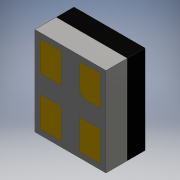
# Autodesk Inventor part: LXDC2HN18A-097
Saved by Autodesk Inventor 2016 (Build 200138000, 138)
## iProperties
Created: 2016-07-07
Part Number: LXDC2HN18A-097
Material: Generic
Document SubType Name: Modeling
Designer: Jonathan
Density: 1 g/cm^3
Appearance: Default
Author: Jonathan
Autodesk Inventor part; units mm, degrees
ref_plane "YZ Plane" through (0, 0, 0) normal (1, 0, 0) x (0, 1, 0)
ref_plane "XZ Plane" through (0, 0, 0) normal (0, 1, 0) x (-1, 0, 0)
ref_plane "XY Plane" through (0, 0, 0) normal (0, 0, 1) x (1, 0, 0)
sketch "Sketch1" plane through (0, 0, 0) normal (0, 1, 0) x (-1, 0, 0)
  line L0 (-1, 1.25) -> (1, 1.25)
  line L1 (1, 1.25) -> (1, -1.25)
  line L2 (1, -1.25) -> (-1, -1.25)
  line L3 (-1, -1.25) -> (-1, 1.25)
  line L4 (-1, 1.25) -> (1, -1.25) construction
  line L5 (1, 1.25) -> (-1, -1.25) construction
  point P0 (0, 0)
  dimension "d0" = 2
  dimension "d1" = 2.5
  constraints: 12 end point, 2 midpoint, 2 parallel, 1 horizontal, 1 perpendicular
  measures "d0" distance of L1.end L2.end
  measures "d1" distance of L0.end L1.end
extrude "Extrusion1" add sketch "Sketch1" along normal blind 0.6
sketch "Sketch2" plane through (0, 0.6, 0) normal (0, 1, 0) x (1, 0, 0)
  line L0 (-1, 1.25) -> (-1, -1.25) projected
  line L1 (-1, -1.25) -> (1, -1.25) projected
  line L2 (1, -1.25) -> (1, 1.25) projected
  line L3 (1, 1.25) -> (-1, 1.25) projected
  point P0 (0, 0)
extrude "Extrusion2" add sketch "Sketch2" along normal blind 0.5 separate body
sketch "Sketch3" plane through (0, 0, 0) normal (0, -1, 0) x (1, 0, 0)
  line L0 (0.85, 1.1) -> (0.25, 1.1)
  line L1 (0.25, 1.1) -> (0.25, 0.3914)
  line L2 (0.3914, 0.25) -> (0.85, 0.25)
  line L3 (0.85, 0.25) -> (0.85, 1.1)
  line L4 (-0.25, 1.1) -> (-0.85, 1.1)
  line L5 (-0.85, 1.1) -> (-0.85, 0.25)
  line L6 (-0.85, 0.25) -> (-0.25, 0.25)
  line L7 (-0.25, 0.25) -> (-0.25, 1.1)
  line L8 (-0.25, -0.25) -> (-0.85, -0.25)
  line L9 (-0.85, -0.25) -> (-0.85, -1.1)
  line L10 (-0.85, -1.1) -> (-0.25, -1.1)
  line L11 (-0.25, -1.1) -> (-0.25, -0.25)
  line L12 (0.85, -0.25) -> (0.25, -0.25)
  line L13 (0.25, -0.25) -> (0.25, -1.1)
  line L14 (0.25, -1.1) -> (0.85, -1.1)
  line L15 (0.85, -1.1) -> (0.85, -0.25)
  line L16 (0.3914, 0.25) -> (0.25, 0.3914)
  line L17 (1, 1.25) -> (-1, 1.25) projected
  line L18 (-1, 1.25) -> (-1, -1.25) projected
  line L19 (-1, -1.25) -> (1, -1.25) projected
  line L20 (1, -1.25) -> (1, 1.25) projected
  point P0 (0, 0)
  dimension "d6" = 0.15
  dimension "d7" = 0.15
  dimension "d8" = 0.15
  dimension "d9" = 0.15
  dimension "d10" = 0.15
  dimension "d11" = 0.15
  dimension "d12" = 0.15
  dimension "d13" = 0.85
  dimension "d14" = 0.85
  dimension "d15" = 0.85
  dimension "d16" = 0.85
  dimension "d17" = 0.6
  dimension "d18" = 0.6
  dimension "d19" = 0.2
  dimension "d20" = 135
  constraints: 34 end point, 8 parallel, 4 horizontal, 4 perpendicular, 3 point on line
  measures "d6" distance between parallel lines of L17 L4
  measures "d7" distance between parallel lines of L18 L5
  measures "d8" distance between parallel lines of L18 L9
  measures "d9" distance between parallel lines of L19 L10
  measures "d10" distance between parallel lines of L19 L14
  measures "d11" distance between parallel lines of L20 L15
  measures "d12" distance between parallel lines of L17 L0
  measures "d13" distance of L2.end L0.start
  measures "d14" distance of L6.end L4.start
  measures "d15" distance of L14.end L12.start
  measures "d16" distance of L10.end L8.start
  measures "d17" distance of L9.end L10.end
  measures "d18" distance of L13.end L14.end
  measures "d19" distance of L2.start L1.end
  measures "d20" angle of L16 L2
extrude "Extrusion3" cut sketch "Sketch3" against normal blind 0.01 contours L3 L2 L16 L1 L0 | L7 L6 L5 L4 | L11 L10 L9 L8 | L15 L14 L13 L12 bodies 1
extrude "Extrusion4" add sketch "Sketch3" against normal blind 0.01 separate body contours L3 L2 L16 L1 L0 | L7 L6 L5 L4 | L11 L10 L9 L8 | L15 L14 L13 L12
sketch "Sketch4" plane through (0, 1.1, 0) normal (0, 1, 0) x (1, 0, 0)
  line L0 (0.45, -0.95) -> (0.7, -0.95)
  line L1 (0.7, -0.95) -> (0.7, -0.45)
  line L2 (0.7, -0.45) -> (0.45, -0.45)
  line L3 (0.45, -0.45) -> (0.45, -0.95)
  line L4 (1, -1.25) -> (1, 1.25) projected
  line L5 (-1, -1.25) -> (1, -1.25) projected
  point P0 (0, 0)
  dimension "d25" = 0.3
  dimension "d26" = 0.3
  dimension "d27" = 0.5
  dimension "d28" = 0.25
  constraints: 8 end point, 2 parallel, 1 horizontal, 1 perpendicular
  measures "d25" distance between parallel lines of L4 L1
  measures "d26" distance between parallel lines of L5 L0
  measures "d27" distance of L2.end L0.start
  measures "d28" distance of L1.end L2.end
extrude "Extrusion5" cut sketch "Sketch4" against normal blind 0.05 bodies 2
body "Solid1"
body "Solid2"
body "Solid3"
